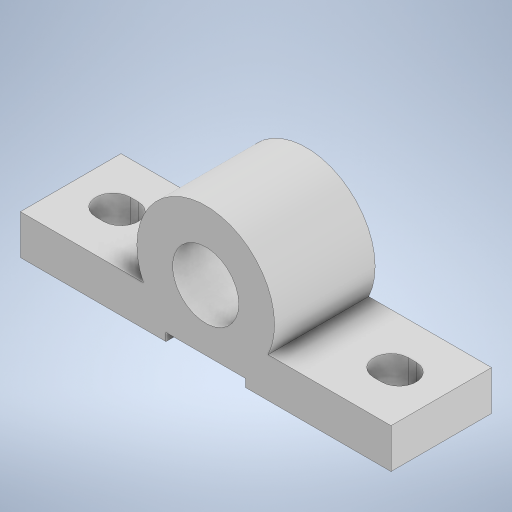
# Autodesk Inventor part: Подшипник с лапками
Saved by Autodesk Inventor 2023 (Build 270158000, 158)
## iProperties
Created: 2022-05-17
Part Number: Подшипник с лапками
Material: Типовые
Document SubType Name: Modeling
Designer: avkap
Density: 1 g/cm^3
Appearance: По умолчанию
Author: avkap
Autodesk Inventor part; units mm, degrees
ref_plane "YZ Plane" through (0, 0, 0) normal (1, 0, 0) x (0, 1, 0)
ref_plane "XZ Plane" through (0, 0, 0) normal (0, 1, 0) x (-1, 0, 0)
ref_plane "XY Plane" through (0, 0, 0) normal (0, 0, 1) x (1, 0, 0)
sketch "Эскиз1" plane through (0, 0, 0) normal (0, 0, 1) x (1, 0, 0)
  circle A0 centre (0, 0) radius 12.5
  circle A1 centre (0, 0) radius 26
  line L0 (0, -26) -> (-70, -26)
  line L1 (-70, -26) -> (70, -26)
  line L2 (70, -26) -> (70, -11)
  line L3 (70, -11) -> (-70, -11)
  line L4 (-70, -11) -> (-70, -26)
  line L5 (0, -26) -> (-15, -26)
  line L6 (-15, -26) -> (-15, -23)
  line L7 (-15, -23) -> (15, -23)
  line L8 (15, -23) -> (15, -26)
  point P0 (23.5584, -11)
  point P1 (-23.5584, -11)
  dimension "d1" = 52
  dimension "d0" = 25
  dimension "d2" = 70
  dimension "d5" = 15
  dimension "d6" = 15
  dimension "d7" = 3
  dimension "d8" = 30
  constraints: 18 end point, 3 horizontal, 2 coincident, 2 parallel, 2 point on line, 2 vertical, 1 centre point, 1 perpendicular, 3 other
  measures "d0" diameter of A0
  measures "d2" distance of L0.start L0.end
  measures "d5" distance of L1.end L2.end
  measures "d6" distance of L0.start L5.end
  measures "d7" distance of L5.end L6.end
  measures "d8" distance of L6.end L7.end
extrude "Выдавливание1" add sketch "Эскиз1" along normal blind 38 contours A0 L3 A1 | A0 L3 A1 L7 | A1 L7 L6 L0 L4 L3 | L3 L2 L1 L8 L7 A1
sketch "Эскиз2" plane through (-70, -11, 0) normal (0, 1, 0) x (1, 0, 0)
  line L0 (0, 0) -> (0, -38) projected
  line L1 (85, 0) -> (140, 0) projected
  line L2 (0, -38) -> (140, -38)
  line L3 (140, -38) -> (140, 0)
  line L4 (140, 0) -> (0, 0)
  line L5 (0, 0) -> (0, -38)
  line L6 (70, 0) -> (70, -38)
  line L7 (70, -19) -> (122.5, -19)
  line L8 (122.5, -19) -> (17.5, -19)
  line L9 (17.5, -19) -> (19, -19)
  line L10 (19, -19) -> (16, -19)
  arc A0 (16, -12.5) -> (16, -25.5) centre (16, -19) ccw
  arc A1 (19, -25.5) -> (19, -12.5) centre (19, -19) ccw
  line L11 (16, -25.5) -> (19, -25.5)
  line L12 (19, -12.5) -> (16, -12.5)
  line L13 (122.5, -19) -> (121, -19)
  line L14 (121, -19) -> (124, -19)
  arc A2 (124, -25.5) -> (124, -12.5) centre (124, -19) ccw
  arc A3 (121, -12.5) -> (121, -25.5) centre (121, -19) ccw
  line L15 (121, -25.5) -> (124, -25.5)
  line L16 (121, -12.5) -> (124, -12.5)
  dimension "d11" = 52.5
  dimension "d12" = 105
  dimension "d13" = 1.5
  dimension "d14" = 3
  dimension "d15" = 13
  dimension "d16" = 1.5
  dimension "d17" = 3
  constraints: 30 end point, 8 point on circle, 5 point on line, 5 tangent, 4 centre point, 4 coincident, 3 horizontal, 3 parallel, 2 midpoint, 1 perpendicular
  measures "d11" distance of L7.start L7.end
  measures "d12" distance of L7.end L8.end
  measures "d13" distance of L8.end L9.end
  measures "d14" distance of L9.end L10.end
  measures "d15" diameter of A0
  measures "d16" distance of L7.end L13.end
  measures "d17" distance of L13.end L14.end
extrude "Выдавливание2" cut sketch "Эскиз2" against normal blind 53.75 contours L12 A1 L11 A0 | L15 A3 L16 A2
